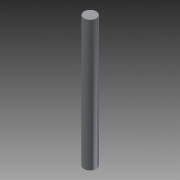
# Autodesk Inventor part: LaserMountPole2
Saved by Autodesk Inventor 2011 (Build 150239000, 239)
## iProperties
Created: 2010-07-18
Part Number: LaserMountPole2
Document SubType Name: Modeling
Designer: abarry
Density: 1 g/cm^3
Author: abarry
Autodesk Inventor part; units mm, degrees
ref_plane "YZ Plane" through (0, 0, 0) normal (1, 0, 0) x (0, 1, 0)
ref_plane "XZ Plane" through (0, 0, 0) normal (0, 1, 0) x (-1, 0, 0)
ref_plane "XY Plane" through (0, 0, 0) normal (0, 0, 1) x (1, 0, 0)
sketch "Sketch1" plane through (0, 0, 0) normal (0, 0, 1) x (1, 0, 0)
  circle A0 centre (0, 0) radius 1.65
  dimension "d0" = 3.3
  dimension "d0" = 3.3
  constraints: 1 centre point, 1 coincident
  measures "d0" diameter of A0
extrude "Extrusion1" add sketch "Sketch1" along normal blind 35
body "Solid1"
